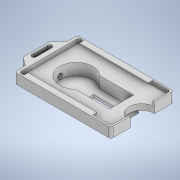
# Autodesk Inventor part: badge
Saved by Autodesk Inventor 2020 (Build 240168000, 168)
## iProperties
Created: 2019-12-22
Part Number: badge
Material: Generic
Document SubType Name: Modeling
Designer: user
Density: 1 g/cm^3
Appearance: Default
Author: user
## iProperties of the stored document _3DPrint.ipt
Created: 2019-12-23
Part Number: _3DPrint
Material: Generic
Document SubType Name: Modeling
Designer: user
Density: 1 g/cm^3
Appearance: Default
Author: user
Autodesk Inventor part; units mm, degrees
ref_plane "YZ Plane" through (0, 0, 0) normal (1, 0, 0) x (0, 1, 0)
ref_plane "XZ Plane" through (0, 0, 0) normal (0, 1, 0) x (-1, 0, 0)
ref_plane "XY Plane" through (0, 0, 0) normal (0, 0, 1) x (1, 0, 0)
sketch "Sketch1" plane through (0, 0, 0) normal (0, 1, 0) x (-1, 0, 0)
  line L0 (9.4719, 24.7859) -> (-76.3174, 24.7859)
  line L1 (-76.3231, -34.0141) -> (9.4769, -34.0141)
  line L2 (11.4719, 14.7859) -> (18.652, 9.5722)
  line L3 (19.4769, 7.9539) -> (19.4769, -15.1857)
  line L4 (18.8911, -16.5999) -> (11.4769, -24.0141)
  line L5 (13.4769, 2.7859) -> (13.4769, -12.0141)
  line L6 (17.4769, -12.0141) -> (17.4769, 2.7859)
  arc A0 (15.4769, -14.0141) -> (17.4769, -12.0141) centre (15.4769, -12.0141) ccw
  arc A1 (13.4769, -12.0141) -> (15.4769, -14.0141) centre (15.4769, -12.0141) ccw
  arc A2 (15.4769, 4.7859) -> (13.4769, 2.7859) centre (15.4769, 2.7859) ccw
  arc A3 (17.4769, 2.7859) -> (15.4769, 4.7859) centre (15.4769, 2.7859) ccw
  arc A4 (-78.3231, -16.0141) -> (-78.3174, 6.7859) centre (-77.6191, -4.6143) ccw
  circle A5 centre (-16.6184, -4.6141) radius 18.5
  line L7 (-61.9161, 7.6359) -> (-61.9161, -16.8641)
  line L8 (-59.9161, -18.8641) -> (-28.4161, -18.8641)
  line L9 (-28.4161, 9.6359) -> (-59.9161, 9.6359)
  arc A6 (-61.9161, -16.8641) -> (-59.9161, -18.8641) centre (-59.9161, -16.8641) ccw
  arc A7 (-59.9161, 9.6359) -> (-61.9161, 7.6359) centre (-59.9161, 7.6359) ccw
  line L10 (-28.8161, -0.3641) -> (-54.3161, -0.3641)
  line L11 (-54.3161, -0.3641) -> (-54.3161, -8.8641)
  line L12 (-54.3161, -8.8641) -> (-28.8161, -8.8641)
  line L13 (-28.8161, -8.8641) -> (-28.8161, -0.3641)
  line L14 (-78.3174, 6.7859) -> (-78.3174, 22.7859)
  line L15 (-78.3231, -16.0141) -> (-78.3231, -32.0141)
  line L16 (6.9737, 23.2859) -> (-74.8231, 23.2859)
  line L17 (-74.8231, -32.5141) -> (6.9737, -32.5141)
  line L18 (8.9737, -30.5141) -> (8.9737, 21.2859)
  line L19 (-76.8231, 21.2859) -> (-76.8231, 6.7795)
  line L20 (-76.8231, -30.5141) -> (-76.8231, -16.008)
  line L21 (11.4719, 22.7859) -> (11.4719, 14.7859)
  line L22 (11.4769, -24.0141) -> (11.4769, -32.0141)
  arc A8 (-78.3231, -32.0141) -> (-76.3231, -34.0141) centre (-76.3231, -32.0141) ccw
  arc A9 (-76.8231, -30.5141) -> (-74.8231, -32.5141) centre (-74.8231, -30.5141) ccw
  arc A10 (-74.8231, 23.2859) -> (-76.8231, 21.2859) centre (-74.8231, 21.2859) ccw
  arc A11 (-76.3174, 24.7859) -> (-78.3174, 22.7859) centre (-76.3174, 22.7859) ccw
  arc A12 (11.4719, 22.7859) -> (9.4719, 24.7859) centre (9.4719, 22.7859) ccw
  arc A13 (8.9737, 21.2859) -> (6.9737, 23.2859) centre (6.9737, 21.2859) ccw
  arc A14 (6.9737, -32.5141) -> (8.9737, -30.5141) centre (6.9737, -30.5141) ccw
  arc A15 (9.4769, -34.0141) -> (11.4769, -32.0141) centre (9.4769, -32.0141) ccw
  arc A16 (18.8911, -16.5999) -> (19.4769, -15.1857) centre (17.4769, -15.1857) ccw
  arc A17 (19.4769, 7.9539) -> (18.652, 9.5722) centre (17.4769, 7.9539) ccw
  point P0 (0, 0)
  point P1 (11.4719, 24.7859)
  point P2 (-78.3231, -34.0141)
  point P3 (-78.3174, 24.7859)
  point P4 (11.4769, -34.0141)
  point P5 (19.4769, -16.0141)
  point P6 (-61.9161, -18.8641)
  point P7 (15.4769, 4.7859)
  point P8 (15.4769, -14.0141)
  dimension "d1" = 89.8
  dimension "d2" = 8
  dimension "d11" = 10
  dimension "d12" = 10
  dimension "d14" = 2
  dimension "d16" = 2
  dimension "d17" = 2
  dimension "d19" = 18
  dimension "d20" = 37
  dimension "d23" = 22.8
  dimension "d24" = 33.5
  dimension "d25" = 28.5
  dimension "d26" = 2
  dimension "d28" = 10
  dimension "d32" = 10
  dimension "d33" = 7.6
  dimension "d34" = 25.5
  dimension "d36" = 1.5
  dimension "d37" = 1.5
  dimension "d40" = 1.5
  dimension "d41" = 2
  dimension "d84" = 55.8
  dimension "d85" = 10
  dimension "d86" = 10
  dimension "d87" = 27.9
  dimension "d88" = 27.9
  dimension "d89" = 18
  constraints: 46 end point, 38 point on circle, 28 tangent, 18 centre point, 13 point on line, 12 equal radius, 8 parallel, 5 vertical, 3 horizontal, 3 perpendicular, 2 coincident, 8 other
  measures "d1" distance of point (-78.323, -34.014) point (11.477, -34.014)
  measures "d2" horizontal distance of point (19.477, -16.014) L4.end
  measures "d14" distance between parallel lines of L3 L6
  measures "d16" radius of A0
  measures "d17" radius of A1
  measures "d19" distance of point (-78.317, 24.786) L14.start
  measures "d20" diameter of A5
  measures "d23" distance of L15.start L14.start
  measures "d24" distance of point (-61.916, -18.864) L8.end
  measures "d25" distance of L8.end L9.start
  measures "d26" radius of A6
  measures "d28" distance between parallel lines of L8 L12
  measures "d32" distance between parallel lines of L10 L9
  measures "d33" distance between parallel lines of L7 L11
  measures "d34" distance of L11.end L12.end
  measures "d36" distance between parallel lines of L0 L16
  measures "d37" distance between parallel lines of L1 L17
  measures "d40" distance between parallel lines of L15 L20
  measures "d41" radius of A8
  measures "d84" distance between parallel lines of L17 L16
  measures "d85" distance of point (11.472, 24.786) L2.start
  measures "d86" distance of point (11.477, -34.014) L4.end
  measures "d87" distance from line of A5.centre L17
  measures "d88" distance from line of L16 A5.centre
  measures "d89" distance of L15.start point (-78.323, -34.014)
extrude "OutsideFrame_Ex" add sketch "Sketch1" along normal blind 9.4 contours A12 L21 L2 A17 L3 A16 L4 L22 A15 L1 A8 L15 A4 L20 A9 L17 A14 L18 A13 L16 A10 L19 L14 A11 L0
extrude "CardRidge" add sketch "Sketch1" along normal blind 5.4 contours L19 A10 L16 A13 L18 A14 L17 A9 L20 A4
extrude "TokenBuffer" add sketch "Sketch1" against normal blind 8.6 contours A5 L12 L13 L10 | A5 L10 L11 L12 L8 A6 L7 A7 L9 picked at (-18.5835, -4.6141)
sketch "Sketch4" plane through (0, 0, 0) normal (0, 1, 0) x (1, 0, 0)
  arc A0 (28.4161, 18.8641) -> (28.4161, -9.6359) centre (16.6184, 4.6141) ccw projected
  circle A1 centre (16.6184, 4.6141) radius 15.5
  line L0 (27.2808, -6.6359) -> (58.9161, -6.6359)
  line L1 (58.9161, -6.6359) -> (58.9161, 15.8641)
  line L2 (58.9161, 15.8641) -> (27.2808, 15.8641)
  line L3 (27.2808, 15.8641) -> (27.2808, -6.6359)
  line L4 (59.9161, -9.6359) -> (28.4161, -9.6359) projected
  line L5 (28.4161, 18.8641) -> (59.9161, 18.8641) projected
  line L6 (61.9161, 16.8641) -> (61.9161, -7.6359) projected
  point P0 (0, 0)
  point P1 (27.2808, 15.8641)
  point P2 (27.2808, 15.8641)
  dimension "d56" = 3
  dimension "d57" = 3
  dimension "d58" = 3
  dimension "d59" = 3
  constraints: 8 end point, 2 parallel, 1 coincident, 1 horizontal, 1 perpendicular, 3 other
  measures "d57" distance between parallel lines of L4 L0
  measures "d58" distance between parallel lines of L5 L2
  measures "d59" distance between parallel lines of L6 L1
extrude "TokenCut" cut sketch "Sketch4" against normal blind 5.6
sketch "Sketch5" plane through (74.8231, 9.4, 23.2859) normal (0, 0, -1) x (-1, 0, 0)
  line L0 (-2, 0) -> (0, 0) projected
  line L1 (79.2968, 0) -> (79.2968, -1)
  line L2 (0, 0) -> (81.7968, 0) projected
  line L3 (15, 0) -> (79.2968, 0)
  line L4 (79.2968, 0) -> (79.2968, -1)
  line L5 (79.2968, -1) -> (15, -1)
  line L6 (15, -1) -> (15, 0)
  line L7 (0, -4) -> (0, 0) projected
  line L8 (81.7968, -4) -> (81.7968, 0) projected
  line L9 (0, -4) -> (81.7968, -4) projected
  point P0 (74.8231, -9.4)
  dimension "d65" = 15
  dimension "d66" = 2.5
  dimension "d67" = 1
  constraints: 10 end point, 2 parallel, 1 horizontal, 1 perpendicular, 1 point on line
  measures "d65" distance between parallel lines of L7 L6
  measures "d66" distance between parallel lines of L8 L1
  measures "d67" distance between parallel lines of L5 L2
extrude "LeftSlider" add sketch "Sketch5" along normal blind 4 contours L1 L5 L6 L2
sketch "Sketch6" plane through (-6.9737, 9.4, -32.5141) normal (0, 0, 1) x (1, 0, 0)
  line L0 (83.2968, 0) -> (-2.5032, 0) projected
  line L1 (2.5, 0) -> (66.7968, 0)
  line L2 (66.7968, 0) -> (66.7968, -1)
  line L3 (66.7968, -1) -> (2.5, -1)
  line L4 (2.5, -1) -> (2.5, 0)
  line L5 (0, -4) -> (0, 0) projected
  line L6 (81.7968, -4) -> (81.7968, 0) projected
  point P0 (6.9737, -9.4)
  dimension "d71" = 2.5
  dimension "d72" = 15
  dimension "d73" = 1
  constraints: 8 end point, 2 parallel, 1 horizontal, 1 perpendicular, 1 point on line
  measures "d71" distance between parallel lines of L5 L4
  measures "d72" distance between parallel lines of L6 L2
  measures "d73" distance between parallel lines of L3 L0
extrude "RightSlider" add sketch "Sketch6" along normal blind 4
sketch "Sketch12" plane through (0, 0, 0) normal (0, 1, 0) x (1, 0, 0)
  arc A0 (27.2808, 15.8641) -> (27.2808, -6.6359) centre (16.6184, 4.6141) ccw projected
  circle A1 centre (16.6184, 4.6141) radius 15.5
  circle A2 centre (16.6184, 4.6141) radius 18.5
  line L0 (59.9161, -9.6359) -> (28.4161, -9.6359) projected
  line L1 (28.4161, -9.6359) -> (59.9161, -9.6359)
  line L2 (61.9161, 16.8641) -> (61.9161, -7.6359) projected
  arc A3 (59.9161, -9.6359) -> (61.9161, -7.6359) centre (59.9161, -7.6359) ccw
  line L3 (58.9161, -6.6359) -> (27.2808, -6.6359) projected
  line L4 (27.2808, -6.6359) -> (58.9161, -6.6359)
  line L5 (58.9161, 15.8641) -> (58.9161, -6.6359) projected
  line L6 (58.9161, -6.6359) -> (58.9161, 15.8641)
  line L7 (27.2808, 15.8641) -> (58.9161, 15.8641) projected
  line L8 (58.9161, 15.8641) -> (27.2808, 15.8641)
  line L9 (61.9161, -7.6359) -> (62.3594, 16.8641)
  line L10 (61.9161, 16.8641) -> (61.9161, -7.6359) projected
  line L11 (61.9161, -7.6359) -> (61.9161, 16.8641)
  line L12 (28.4161, 18.8641) -> (59.9161, 18.8641) projected
  arc A4 (61.9161, 16.8641) -> (59.9161, 18.8641) centre (59.9161, 16.8641) ccw
  line L13 (59.9161, 18.8641) -> (28.4161, 18.8641)
  point P0 (0, 0)
  point P1 (31.3047, 15.8641)
  point P2 (31.3047, -6.6359)
  constraints: 14 end point, 4 centre point, 4 point on circle, 2 coincident, 2 horizontal, 2 perpendicular, 1 collinear, 1 tangent
extrude "Extrusion13" add sketch "Sketch12" along normal blind 5.4 contours A2 L12 A4 L2 A3 L0 L3 L5 L7
extrude "Extrusion14" add sketch "Sketch12" along normal blind 5.4 contours A0 L3 A2 L7
sketch "Sketch13" plane through (58.9161, -5.6, -15.8641) normal (-1, 0, 0) x (0, 0, 1)
  line L0 (22.5, 11) -> (22.5, 0) projected
  line L1 (0, 11) -> (0, 0) projected
  line L2 (0, 0) -> (22.5, 0) projected
  point P0 (15.8641, 5.6)
  point P1 (11.25, 2.8786)
  dimension "d101" = 11.25
  dimension "d102" = 11.25
  dimension "d103" = 2.8786
  measures "d101" distance from line of L0 point (11.25, 2.879)
  measures "d102" distance from line of L1 point (11.25, 2.879)
  measures "d103" distance from line of L2 point (11.25, 2.879)
hole "Hole1" at (58.9161, -2.7214, -4.6141) direction (-1, 0, 0) diameter 5 end through all
equation "\"d12\" = d11"
equation "\"d86\" = d85"
equation "\"d87\" = d88"
equation "\"d89\" = d19"
body "Solid3"
